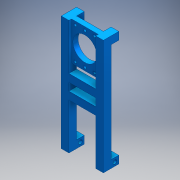
# Autodesk Inventor part: framesideRight
Saved by Autodesk Inventor 2016 (Build 200138000, 138)
## iProperties
Created: 2016-05-18
Part Number: framesideRight
Material: ABS Plastic
Document SubType Name: Modeling
Designer: hesaon
Density: 1.06 g/cm^3
Appearance: Smooth - White
Author: hesaon
Autodesk Inventor part; units mm, degrees
ref_plane "YZ Plane" through (0, 0, 0) normal (1, 0, 0) x (0, 1, 0)
ref_plane "XZ Plane" through (0, 0, 0) normal (0, 1, 0) x (-1, 0, 0)
ref_plane "XY Plane" through (0, 0, 0) normal (0, 0, 1) x (1, 0, 0)
sketch "Sketch1" plane through (0, 0, 0) normal (0, 1, 0) x (-1, 0, 0)
  line L0 (0, 0) -> (66, 0)
  line L1 (66, 0) -> (66, -180)
  line L2 (66, -180) -> (0, -180)
  line L3 (0, -180) -> (0, 0)
  line L4 (54, -12) -> (12, -12)
  line L5 (12, -168) -> (54, -168)
  line L6 (54, -72) -> (12, -72)
  line L7 (54, -84) -> (12, -84)
  line L8 (54, -168) -> (54, -84)
  line L9 (54, -72) -> (54, -12)
  line L10 (12, -12) -> (12, -72)
  line L11 (12, -84) -> (12, -168)
  dimension "d0" = 66
  dimension "d1" = 180
  dimension "d3" = 42
  dimension "d4" = 12
  dimension "d5" = 12
  dimension "d6" = 60
  dimension "d7" = 12
  dimension "d8" = 12
  dimension "d9" = 12
  constraints: 24 end point, 7 perpendicular, 6 parallel, 2 horizontal, 1 collinear
  measures "d0" distance of L1.end L2.end
  measures "d1" distance of L0.end L1.end
  measures "d3" distance of L5.start L5.end
  measures "d4" distance from line of L2 L5.start
  measures "d5" distance from line of L1 L5.end
  measures "d6" distance of L4.end L6.end
  measures "d7" distance of L7.end L6.end
  measures "d8" distance between parallel lines of L0 L4
  measures "d9" distance from line of L3 L4.end
extrude "Extrusion1" add sketch "Sketch1" along normal blind 12
sketch "Sketch4" plane through (0, 0, 0) normal (0, -1, 0) x (1, 0, 0)
  line L0 (-66, 0) -> (-66, -180) projected
  line L1 (-26, 0) -> (-12, 0)
  line L2 (-12, 0) -> (-12, -12)
  line L3 (-12, -12) -> (-26, -12)
  line L4 (-26, -12) -> (-26, 0)
  line L5 (-54, 0) -> (-40, 0)
  line L6 (-40, 0) -> (-40, -12)
  line L7 (-40, -12) -> (-54, -12)
  line L8 (-54, -12) -> (-54, 0)
  point P0 (-54, -12)
  point P1 (-12, -12)
  dimension "d87" = 14
  dimension "d88" = 12
  dimension "d89" = 14
  dimension "d90" = 12
  constraints: 16 end point, 4 parallel, 2 coincident, 2 horizontal, 2 perpendicular
  measures "d87" distance of L2.end L3.end
  measures "d88" distance of L1.end L2.end
  measures "d89" distance of L6.end L7.end
  measures "d90" distance of L5.end L6.end
extrude "Extrusion5" cut sketch "Sketch4" against normal up to next
sketch "Sketch6" plane through (0, 0, 0) normal (0, -1, 0) x (1, 0, 0)
  line L0 (-54, -84) -> (-54, -168) projected
  line L1 (-54, -168) -> (-12, -168)
  line L2 (-12, -168) -> (-12, -180)
  line L3 (-12, -180) -> (-54, -180)
  line L4 (-54, -180) -> (-54, -168)
  point P0 (0, 0)
  dimension "d100" = 42
  dimension "d101" = 12
  constraints: 8 end point, 2 parallel, 1 horizontal, 1 perpendicular
  measures "d100" distance of L2.end L3.end
  measures "d101" distance of L1.end L2.end
extrude "Extrusion7" cut sketch "Sketch6" against normal up to next
sketch "Sketch8" plane through (0, 0, 0) normal (0, -1, 0) x (1, 0, 0)
  line L0 (-54, -84) -> (-54, -180) projected
  line L1 (-54, -96) -> (-12, -96)
  line L2 (-12, -84) -> (-12, -180) projected
  line L3 (-12, -108) -> (-54, -108)
  point P0 (0, 0)
  dimension "d110" = 12
  dimension "d111" = 12
  constraints: 4 end point, 4 point on line, 1 horizontal, 1 parallel
  measures "d110" distance of L0.start L1.start
  measures "d111" distance of L3.end L1.start
extrude "Extrusion9" add sketch "Sketch8" against normal blind 12
sketch "Sketch9" plane through (-12, 0, -108) normal (0, 0, -1) x (-1, 0, 0)
  circle A0 centre (7, 6) radius 2.5
  line L0 (42, 0) -> (0, 0) projected
  line L1 (0, 0) -> (0, 12) projected
  circle A1 centre (24, 6) radius 2.5
  line L2 (42, 12) -> (42, 0) projected
  point P0 (-12, 0)
  dimension "d114" = 5
  dimension "d115" = 6
  dimension "d116" = 7
  dimension "d117" = 5
  dimension "d118" = 6
  dimension "d124" = 17
  constraints: 2 centre point
  measures "d114" diameter of A0
  measures "d115" distance from line of L0 A0.centre
  measures "d116" distance from line of L1 A0.centre
  measures "d117" diameter of A1
  measures "d118" distance from line of L0 A1.centre
  measures "d124" distance of A1.centre A0.centre
extrude "Extrusion10" cut sketch "Sketch9" against normal blind 6
fillet "Fillet1" radius 2.5 1 edges at (-16.5, 6, -102)
fillet "Fillet2" radius 2.5 1 edges at (-33.5, 6, -102)
sketch "Sketch13" plane through (0, 12, 0) normal (0, 1, 0) x (1, 0, 0)
  line L0 (0, 180) -> (-12, 180) projected
  line L1 (0, 180) -> (-12, 180)
  line L2 (-12, 180) -> (-12, 168)
  line L3 (-12, 168) -> (0, 168)
  line L4 (0, 168) -> (0, 180)
  line L5 (-66, 180) -> (-54, 180) projected
  line L6 (-54, 180) -> (-66, 180)
  line L7 (-66, 180) -> (-66, 168)
  line L8 (-66, 168) -> (-54, 168)
  line L9 (-54, 168) -> (-54, 180)
  point P0 (0, 0)
  dimension "d136" = 12
  dimension "d137" = 12
  dimension "d138" = 12
  dimension "d139" = 12
  constraints: 16 end point, 4 parallel, 2 horizontal, 2 perpendicular
  measures "d136" distance of L3.end L2.end
  measures "d137" distance of L2.end L1.end
  measures "d138" distance of L8.end L7.end
  measures "d139" distance of L7.end L6.end
extrude "Extrusion13" add sketch "Sketch13" along normal blind 12
sketch "Sketch14" plane through (0, 0, 0) normal (1, 0, 0) x (0, 0, -1)
  circle A0 centre (174, 18) radius 3
  line L0 (168, 12) -> (168, 24) projected
  line L1 (168, 24) -> (180, 24) projected
  point P0 (0, 0)
  dimension "d142" = 6
  dimension "d143" = 6
  dimension "d144" = 6
  constraints: 1 centre point
  measures "d142" diameter of A0
  measures "d143" distance from line of L0 A0.centre
  measures "d144" distance from line of L1 A0.centre
extrude "Extrusion14" cut sketch "Sketch14" against normal blind 66
sketch "Sketch15" plane through (0, 12, 0) normal (0, 1, 0) x (1, 0, 0)
  line L0 (0, 0) -> (0, 168) projected
  line L1 (-26, 12) -> (-12, 12) projected
  line L2 (0, 0) -> (-12, 0)
  line L3 (-12, 0) -> (-12, 12)
  line L4 (-12, 12) -> (0, 12)
  line L5 (0, 12) -> (0, 0)
  line L6 (-54, 72) -> (-54, 0) projected
  line L7 (-54, 0) -> (-66, 0)
  line L8 (-66, 0) -> (-66, 12)
  line L9 (-66, 12) -> (-54, 12)
  line L10 (-54, 12) -> (-54, 0)
  dimension "d147" = 12
  dimension "d148" = 12
  dimension "d149" = 12
  dimension "d150" = 12
  constraints: 16 end point, 4 parallel, 2 horizontal, 2 perpendicular
  measures "d147" distance of L1.end L4.end
  measures "d148" distance of L2.end L1.end
  measures "d149" distance of L8.end L9.end
  measures "d150" distance of L7.end L8.end
extrude "Extrusion15" add sketch "Sketch15" along normal blind 12
sketch "Sketch17" plane through (0, 0, 0) normal (0, -1, 0) x (1, 0, 0)
  line L0 (-40, 0) -> (-40, -12) projected
  line L1 (-26, 0) -> (-40, 0) projected
  line L2 (-40, -12) -> (-26, -12)
  line L3 (-26, -12) -> (-26, 0)
  line L4 (-26, 0) -> (-40, 0)
  line L5 (-40, 0) -> (-40, -12)
  point P0 (0, 0)
  constraints: 8 end point, 2 parallel, 1 horizontal, 1 perpendicular
extrude "Extrusion16" cut sketch "Sketch17" against normal blind 12
sketch "Sketch18" plane through (0, 12, 0) normal (0, 1, 0) x (1, 0, 0)
  line L0 (-12, 0) -> (-12, 72) projected
  line L1 (-12, 0) -> (-54, 0)
  line L2 (-54, 0) -> (-54, 60)
  line L3 (-54, 60) -> (-12, 60)
  line L4 (-12, 60) -> (-12, 0)
  point P0 (0, 0)
  dimension "d155" = 42
  dimension "d156" = 60
  constraints: 8 end point, 2 parallel, 1 horizontal, 1 perpendicular
  measures "d155" distance of L2.end L3.end
  measures "d156" distance from line of L1 L2.end
extrude "Extrusion17" add sketch "Sketch18" against normal blind 8
sketch "Sketch19" plane through (0, 4, 0) normal (0, -1, 0) x (1, 0, 0)
  circle A0 centre (-33, -30) radius 18.75
  line L0 (-54, -72) -> (-54, 0) projected
  line L1 (-12, 0) -> (-54, 0) projected
  circle A1 centre (-33, -5) radius 2.1
  circle A2 centre (-18, -5) radius 2.1
  circle A3 centre (-18, -55) radius 2.1
  circle A4 centre (-33, -55) radius 2.1
  circle A5 centre (-48, -55) radius 2.1
  circle A6 centre (-48, -5) radius 2.1
  line L2 (-54, -60) -> (-12, -60) projected
  point P0 (0, 0)
  dimension "d159" = 37.5
  dimension "d160" = 21
  dimension "d161" = 30
  dimension "d162" = 4.2
  dimension "d163" = 5
  dimension "d164" = 0
  dimension "d165" = 4.2
  dimension "d166" = 4.2
  dimension "d167" = 4.2
  dimension "d168" = 4.2
  dimension "d169" = 4.2
  dimension "d170" = 5
  dimension "d171" = 5
  dimension "d172" = 5
  dimension "d173" = 5
  dimension "d174" = 5
  dimension "d175" = 15
  dimension "d176" = 15
  dimension "d177" = 15
  dimension "d178" = 0
  dimension "d179" = 15
  constraints: 7 centre point
  measures "d159" diameter of A0
  measures "d160" distance from line of L0 A0.centre
  measures "d161" distance from line of L1 A0.centre
  measures "d162" diameter of A1
  measures "d163" distance from line of L1 A1.centre
  measures "d164" horizontal distance of A0.centre A1.centre
  measures "d165" diameter of A2
  measures "d166" diameter of A3
  measures "d167" diameter of A4
  measures "d168" diameter of A5
  measures "d169" diameter of A6
  measures "d170" distance from line of L1 A2.centre
  measures "d171" distance from line of L1 A6.centre
  measures "d172" distance from line of L2 A3.centre
  measures "d173" distance from line of L2 A4.centre
  measures "d174" distance from line of L2 A5.centre
  measures "d175" distance of A2.centre A1.centre
  measures "d176" distance of A1.centre A6.centre
  measures "d177" distance of A4.centre A3.centre
  measures "d178" horizontal distance of A0.centre A4.centre
  measures "d179" distance of A4.centre A5.centre
extrude "Extrusion18" cut sketch "Sketch19" against normal up to next
body "Solid1"
